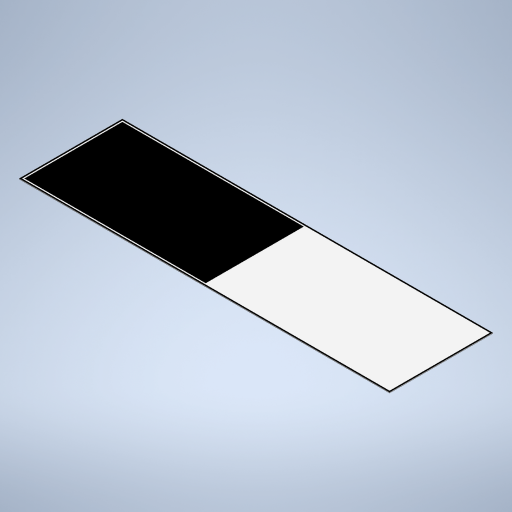
# Autodesk Inventor part: banner
Saved by Autodesk Inventor 2024.1 (Build 281209000, 209)
## iProperties
Created: 2023-11-13
Part Number: banner
Material: Generic
Document SubType Name: Modeling
Designer: ASUS
Density: 1 g/cm^3
Appearance: Default
Author: ASUS
Autodesk Inventor part; units mm, degrees
ref_plane "YZ Plane" through (0, 0, 0) normal (1, 0, 0) x (0, 1, 0)
ref_plane "XZ Plane" through (0, 0, 0) normal (0, 1, 0) x (-1, 0, 0)
ref_plane "XY Plane" through (0, 0, 0) normal (0, 0, 1) x (1, 0, 0)
sketch "Sketch2" plane through (0, 0, 0) normal (0, 1, 0) x (-1, 0, 0)
  line L0 (0, -19812) -> (71120, -19812)
  line L1 (71120, -19812) -> (71120, 0)
  line L2 (71120, 0) -> (0, 0)
  line L3 (0, 0) -> (0, -19812)
  line L4 (70866, -19558) -> (254, -19558)
  line L5 (254, -19558) -> (254, -254)
  line L6 (254, -254) -> (70866, -254)
  line L7 (70866, -254) -> (70866, -19558)
  line L8 (70612, -19304) -> (35814, -19304)
  line L9 (35814, -19304) -> (35814, -508)
  line L10 (35814, -508) -> (70612, -508)
  line L11 (70612, -508) -> (70612, -19304)
  constraints: 24 end point, 6 parallel, 3 perpendicular, 2 horizontal, 3 other
extrude "Extrusion5" add sketch "Sketch2" along normal blind 127 contours L8 L9 L10 L11
extrude "Extrusion6" add sketch "Sketch2" along normal blind 127 separate body contours L4 L5 L6 L7
extrude "Extrusion7" add sketch "Sketch2" along normal blind 127 separate body contours L3 L2 L1 L0
body "Solid5"
body "Solid6"
body "Solid7"
